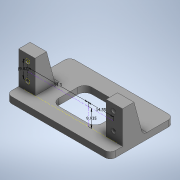
# Autodesk Inventor part: MG996R Attachment Test
Saved by Autodesk Inventor 2020.5 (Build 245400000, 400)
## iProperties
Created: 2023-03-16
Part Number: MG996R Attachment Test
Material: Generic
Document SubType Name: Modeling
Designer: Wes
Density: 1 g/cm^3
Appearance: Default
Author: Wes
Autodesk Inventor part; units mm, degrees
ref_plane "YZ Plane" through (0, 0, 0) normal (1, 0, 0) x (0, 1, 0)
ref_plane "XZ Plane" through (0, 0, 0) normal (0, 1, 0) x (-1, 0, 0)
ref_plane "XY Plane" through (0, 0, 0) normal (0, 0, 1) x (1, 0, 0)
sketch "Base" plane through (0, 0, 0) normal (0, 0, 1) x (1, 0, 0)
  line L0 (0, 0) -> (-36, 0)
  line L1 (-36, 0) -> (-36, 59)
  line L2 (-36, 59) -> (0, 59)
  line L3 (0, 59) -> (0, 0)
  dimension "d0" = 36
  dimension "d1" = 59
  constraints: 8 end point, 2 parallel, 1 horizontal, 1 perpendicular
  measures "d0" distance of L1.end L2.end
  measures "d1" distance of L0.end L1.end
extrude "Extrusion1" add sketch "Base" along normal mid plane 3.5
sketch "Attachment Towers" plane through (0, 0, 1.75) normal (0, 0, 1) x (1, 0, 0)
  line L0 (0, 29.5) -> (-7, 29.5) construction
  line L1 (-7, 29.5) -> (-7, 49.7) construction
  line L2 (-7, 29.5) -> (-7, 9.3) construction
  line L3 (-7, 49.7) -> (-13.5, 49.7)
  line L4 (-13.5, 49.7) -> (-13.5, 59)
  line L5 (-13.5, 59) -> (-7, 59)
  line L6 (-7, 59) -> (-7, 49.7)
  line L7 (-7, 9.3) -> (-13.5, 9.3)
  line L8 (-13.5, 9.3) -> (-13.5, 0)
  line L9 (-13.5, 0) -> (-7, 0)
  line L10 (-7, 0) -> (-7, 9.3)
  dimension "d41" = 7
  dimension "d44" = 40.4
  dimension "d45" = 6.5
  dimension "d46" = 9.3
  constraints: 22 end point, 4 parallel, 3 horizontal, 2 perpendicular, 1 vertical
  measures "d41" distance of L0.start L0.end
  measures "d44" distance of L1.end L2.end
  measures "d45" distance of L4.end L5.end
  measures "d46" distance of L3.end L4.end
extrude "Extrusion3" add sketch "Attachment Towers" along normal blind 18.5
sketch "Screw Holes" plane through (-7, 0, 1.75) normal (1, 0, 0) x (0, 0, -1)
  line L0 (0, 49.7) -> (0, 51.8) construction
  line L1 (0, 51.8) -> (-7.15, 51.8) construction
  circle A0 centre (-5.025, 53.925) radius 2.125 construction
  line L2 (-7.15, 51.8) -> (-7.15, 61.0367) construction
  line L3 (-2.9, 53.925) -> (-16.97, 53.925) construction
  circle A1 centre (-14.845, 53.925) radius 2.125 construction
  line L4 (-16.97, 51.8) -> (-16.97, 61.0367) construction
  circle A2 centre (-14.845, 53.925) radius 1.275
  circle A3 centre (-5.025, 53.925) radius 1.275
  line L5 (0, 29.5) -> (-35.6681, 29.5) construction
  circle A4 centre (-14.845, 5.075) radius 1.275
  circle A5 centre (-5.025, 5.075) radius 1.275
  dimension "d18" = 4.25
  dimension "d15" = 2.1
  dimension "d16" = 7.15
  dimension "d20" = 14.07
  dimension "d21" = 4.25
  dimension "d22" = 2.55
  dimension "d23" = 2.55
  constraints: 12 end point, 5 centre point, 3 horizontal, 2 coincident, 2 point on line, 2 symmetric about line, 2 vertical, 1 horizontal alignment, 1 parallel, 1 tangent, 4 other
  measures "d15" distance of L0.start L0.end
  measures "d16" distance of L0.end L1.end
  measures "d20" distance of L3.start L3.end
  measures "d21" diameter of A1
  measures "d22" diameter of A2
  measures "d23" diameter of A3
extrude "Extrusion4" cut sketch "Screw Holes" against normal blind 4
draft "FaceDraft1" angle 15 pull direction (0, 0, 1) faces at (-13.5, 6.2, 7.9167) (-13.5, 55.9, 7.9167) fixed edges at (-13.5, 4.65, 20.25) (-13.5, 54.35, 20.25)
sketch "Sketch5" plane through (0, 0, 1.75) normal (0, 0, 1) x (1, 0, 0)
  line L0 (-36, 29.5) -> (0, 29.5) construction
  line L1 (-23.4056, 41.836) -> (-12.5944, 41.836)
  line L2 (-8.5944, 37.836) -> (-8.5944, 21.164)
  line L3 (-12.5944, 17.164) -> (-23.4056, 17.164)
  line L4 (-27.4056, 21.164) -> (-27.4056, 37.836)
  line L5 (-27.4056, 41.836) -> (-8.5944, 17.164) construction
  line L6 (-8.5944, 41.836) -> (-27.4056, 17.164) construction
  arc A0 (-27.4056, 21.164) -> (-23.4056, 17.164) centre (-23.4056, 21.164) ccw
  arc A1 (-12.5944, 17.164) -> (-8.5944, 21.164) centre (-12.5944, 21.164) ccw
  arc A2 (-8.5944, 37.836) -> (-12.5944, 41.836) centre (-12.5944, 37.836) ccw
  arc A3 (-23.4056, 41.836) -> (-27.4056, 37.836) centre (-23.4056, 37.836) ccw
  point P0 (-18, 29.5)
  dimension "d47" = 4
  constraints: 14 end point, 8 point on circle, 8 point on line, 8 tangent, 4 centre point, 3 equal radius, 3 midpoint, 2 parallel, 1 horizontal, 1 perpendicular
  measures "d47" radius of A0
extrude "Extrusion5" cut sketch "Sketch5" against normal through all
fillet "Fillet1" radius 3 6 edges at (0, 0, 0) (0, 59, 0) (-36, 59, 0) (-36, 0, 0) (-18.4571, 4.65, 1.75) (-18.4571, 54.35, 1.75)
sketch "Axle Reference" plane through (-7, 0, 1.75) normal (1, 0, 0) x (0, 0, -1)
  circle A0 centre (-14.845, 5.075) radius 1.275 construction
  circle A1 centre (-5.025, 5.075) radius 1.275 construction
  line L0 (-9.935, 5.075) -> (-9.935, 39.375) construction
  line L1 (-9.935, 53.925) -> (-9.935, 39.375) construction
  line L2 (-9.935, 39.375) -> (0, 39.375) construction
  line L3 (0, 56) -> (0, 3) construction
  circle A2 centre (-14.845, 5.075) radius 1.275 construction
  line L4 (-14.845, 5.075) -> (-5.025, 5.075) construction
  point P0 (1.75, 0)
  dimension "d48" = 34.3
  dimension "d49" = 14.55
  dimension "d50" = 9.935
  dimension "d51" = 9.82
  constraints: 8 end point, 2 vertical, 1 coincident, 1 horizontal, 1 point on line
  measures "d48" distance of L0.start L0.end
  measures "d49" distance of L1.start L1.end
  measures "d50" distance of L1.end L2.end
  measures "d51" distance of L4.start L4.end
body "Solid1"
